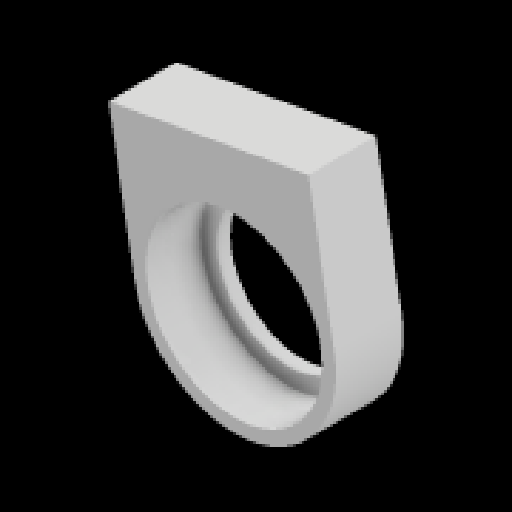
# Autodesk Inventor part: RodBearingMount
Saved by Autodesk Inventor 2025 (Build 290162000, 162)
## iProperties
Created: 2024-11-19
Part Number: RodBearingMount
Material: Generic
Document SubType Name: Modeling
Designer: Trevor
Density: 1 g/cm^3
Appearance: Default
Author: Trevor
Autodesk Inventor part; units mm, degrees
ref_plane "YZ Plane" through (0, 0, 0) normal (1, 0, 0) x (0, 1, 0)
ref_plane "XZ Plane" through (0, 0, 0) normal (0, 1, 0) x (-1, 0, 0)
ref_plane "XY Plane" through (0, 0, 0) normal (0, 0, 1) x (1, 0, 0)
sketch "Sketch1" plane through (0, 0, 0) normal (0, 0, 1) x (1, 0, 0)
  circle A0 centre (0, -6.9891) radius 13 projected
  line L0 (-8.3396, 25.9015) -> (-6.0783, 13.4045)
  line L1 (9.8647, 29.1956) -> (12.126, 16.6985) projected
  line L2 (-201.5028, -9.0509) -> (9.8647, 29.1956) projected
  line L3 (-199.2415, -21.5479) -> (-201.5028, -9.0509) projected
  line L4 (-199.2415, -21.5479) -> (12.126, 16.6985) projected
  line L5 (0, -6.9891) -> (-3.7659, 13.8229) construction
  circle A1 centre (0, -6.9891) radius 15
  line L6 (0, -6.9891) -> (-14.7603, -9.66) construction
  line L7 (-14.7603, -9.66) -> (-18.5262, 11.1521)
  line L8 (0, -6.9891) -> (14.7603, -4.3183) construction
  line L9 (14.7603, -4.3183) -> (10.9944, 16.4937)
  line L10 (10.9944, 16.4937) -> (-18.5262, 11.1521)
  point P0 (0, 0)
  constraints: 14 end point, 4 perpendicular, 3 point on line, 2 point on circle, 1 centre point, 1 collinear, 3 other
ref_plane "Work Plane1" through (-17.5555, -24.5446, -8) normal (0, 0, -1) x (0, 1, 0)
extrude "Extrusion1" add sketch "Sketch1" against normal up to surface (8 mm away) contours L4 L9 A1 L7 | A1
sketch "Sketch2" plane through (0, -6.9891, -8) normal (0, 0, -1) x (-0.9840203, -0.1780561, 0)
  circle A0 centre (0, 0) radius 13 projected
  line L0 (15, 21.15) -> (15, 0) projected
  line L1 (-15, 21.15) -> (15, 21.15) projected
  line L2 (-15, 0) -> (-15, 21.15) projected
  arc A1 (-15, 0) -> (15, 0) centre (0, 0) ccw projected
  circle A2 centre (0, 0) radius 5 projected
  circle A3 centre (0, 0) radius 10.5
  point P0 (-1.2445, 6.8774)
  constraints: 1 centre point, 1 other
extrude "Extrusion2" add sketch "Sketch2" along normal blind 2 contours A0 | L0 A1 L2 L1
ref_plane "Work Plane2" through (-83.7175, -0.6442, 79.375) normal (0.1780561, -0.9840203, 0) x (0, 0, -1)
sketch "Sketch3" plane through (-83.7175, -0.6442, 79.375) normal (0.1780561, -0.9840203, 0) x (0, 0, -1)
  circle A0 centre (-108.5, -103.9) radius 5 projected
  circle A1 centre (108.5, -103.9) radius 5 projected
  circle A2 centre (-108.5, 83.9) radius 5 projected
  circle A3 centre (108.5, 83.9) radius 5 projected
  arc A4 (127, 97.4) -> (122, 102.4) centre (122, 97.4) ccw projected
  line L0 (84.375, 102.4) -> (122, 102.4) projected
  arc A5 (84.375, 102.4) -> (79.375, 97.4) centre (84.375, 97.4) ccw projected
  line L1 (79.375, 97.4) -> (79.375, 25.8) projected
  arc A6 (74.375, 20.8) -> (79.375, 25.8) centre (74.375, 25.8) ccw projected
  line L2 (74.375, 20.8) -> (-74.375, 20.8) projected
  arc A7 (-79.375, 25.8) -> (-74.375, 20.8) centre (-74.375, 25.8) ccw projected
  line L3 (-79.375, 25.8) -> (-79.375, 97.4) projected
  arc A8 (-79.375, 97.4) -> (-84.375, 102.4) centre (-84.375, 97.4) ccw projected
  line L4 (-122, 102.4) -> (-84.375, 102.4) projected
  arc A9 (-122, 102.4) -> (-127, 97.4) centre (-122, 97.4) ccw projected
  line L5 (-127, -117.4) -> (-127, 97.4) projected
  arc A10 (-127, -117.4) -> (-122, -122.4) centre (-122, -117.4) ccw projected
  line L6 (-95, -122.4) -> (-122, -122.4) projected
  arc A11 (-95, -122.4) -> (-90, -117.4) centre (-95, -117.4) ccw projected
  line L7 (-90, -117.4) -> (-90, -47.4) projected
  arc A12 (-85, -42.4) -> (-90, -47.4) centre (-85, -47.4) ccw projected
  line L8 (-85, -42.4) -> (85, -42.4) projected
  arc A13 (90, -47.4) -> (85, -42.4) centre (85, -47.4) ccw projected
  line L9 (90, -47.4) -> (90, -117.4) projected
  arc A14 (90, -117.4) -> (95, -122.4) centre (95, -117.4) ccw projected
  line L10 (122, -122.4) -> (95, -122.4) projected
  arc A15 (122, -122.4) -> (127, -117.4) centre (122, -117.4) ccw projected
  line L11 (127, 97.4) -> (127, -117.4) projected
  line L12 (89.375, 66.25) -> (89.375, 96.25) projected
  line L13 (89.375, 96.25) -> (101.375, 96.25)
  line L14 (101.375, 96.25) -> (101.375, 66.25)
  line L15 (101.375, 66.25) -> (89.375, 66.25)
  line L16 (89.375, 66.25) -> (89.375, 96.25)
  circle A16 centre (95.375, 81.25) radius 2.5
  line L17 (95.375, 96.25) -> (95.375, 66.25)
  circle A17 centre (95.375, 71.25) radius 2.5
  circle A18 centre (95.375, 91.25) radius 2.5
  circle A19 centre (95.375, 81.25) radius 2.5
  line L18 (79.375, 66.25) -> (89.375, 66.25) projected
  point P0 (79.375, 82.4945)
  dimension "d5" = 12
  dimension "d6" = 5
  dimension "d9" = 10
  dimension "d12" = 10
  constraints: 10 end point, 4 centre point, 2 midpoint, 2 parallel, 2 vertical, 1 horizontal, 1 perpendicular, 6 other
  measures "d5" distance of L14.end L15.end
  measures "d6" diameter of A16
  measures "d9" distance of A16.centre A17.centre
  measures "d12" distance of A16.centre A18.centre
extrude "Extrusion3" add sketch "Sketch3" along normal blind 5 contours L12 L13 L17 A18 A16 A17 L15 | L17 A17 A16 A18 L13 L14 L15
body "Solid1"
